SupportWiFiAlpha (Autodesk Fusion 360 design; units mm, degrees)
Autodesk Fusion 360 part; units mm, degrees
note: some values were not read from the file. Chosen so that the rebuilt part matches the saved one: which pieces of a blend or face edit are solid.
sketch "Sketch1" plane through (0, 0, 0) normal (0, 0, 1) x (1, 0, 0)
  line L0 (32.5, -60.9) -> (-32.5, -60.9)
  line L1 (-32.5, -60.9) -> (-32.5, 60.9)
  line L2 (-32.5, 60.9) -> (32.5, 60.9)
  line L3 (32.5, 60.9) -> (32.5, -60.9)
  line L4 (32.5, -60.9) -> (-32.5, 60.9) construction
  line L5 (-32.5, -60.9) -> (32.5, 60.9) construction
  line L6 (0, 0) -> (0, 50.9) construction
  line L7 (-2.1, 52.15) -> (-2.1, 49.65)
  arc A0 (-2.1, 49.65) -> (2.1, 49.65) centre (0, 49.65) ccw
  line L8 (2.1, 49.65) -> (2.1, 52.15)
  arc A1 (2.1, 52.15) -> (-2.1, 52.15) centre (0, 52.15) ccw
  line L9 (0, 52.15) -> (0, 49.65) construction
  line L10 (-32.5, 0) -> (32.5, 0) construction
  arc A2 (-2.1, -52.15) -> (2.1, -52.15) centre (0, -52.15) ccw
  line L11 (-2.1, -52.15) -> (-2.1, -49.65)
  line L12 (2.1, -49.65) -> (2.1, -52.15)
  arc A3 (2.1, -49.65) -> (-2.1, -49.65) centre (0, -49.65) ccw
  line L13 (-31.25, 85) -> (31.25, 85)
  line L14 (31.25, 85) -> (31.25, 0)
  line L15 (31.25, 0) -> (-31.25, 0)
  line L16 (-31.25, 0) -> (-31.25, 85)
  line L17 (-32.5, 60.9) -> (-32.5, 85)
  line L18 (-32.5, 85) -> (-31.25, 85)
  line L19 (32.5, 60.9) -> (32.5, 85)
  line L20 (32.5, 85) -> (31.25, 85)
  line L21 (-32.5, -2) -> (32.5, -2)
  line L22 (-9, 0) -> (9, 0)
  line L23 (9, 0) -> (9, -2)
  line L24 (9, -2) -> (-9, -2)
  line L25 (-9, -2) -> (-9, 0)
  line L26 (0, 85) -> (0, 61) construction
  line L27 (10, 85) -> (-10, 85)
  line L28 (-10, 85) -> (-10, 87)
  line L29 (-10, 87) -> (10, 87)
  line L30 (10, 87) -> (10, 85)
  line L31 (10, 85) -> (-10, 87) construction
  line L32 (-10, 85) -> (10, 87) construction
  line L33 (32.5, 85) -> (-32.5, 85)
  line L34 (-32.5, 85) -> (-32.5, 87)
  line L35 (-32.5, 87) -> (32.5, 87)
  line L36 (32.5, 87) -> (32.5, 85)
  line L37 (32.5, 85) -> (-32.5, 87) construction
  line L38 (-32.5, 85) -> (32.5, 87) construction
  point P0 (0, 50.9)
  point P1 (0, 86)
  point P2 (0, 86)
  dimension "d1" = 121.8
  dimension "d2" = 65
  dimension "d3" = 50.9
  dimension "d4" = 4.2
  dimension "d5" = 2.5
  dimension "d8" = 85
  dimension "d9" = 62.5
  dimension "d10" = 2
  dimension "d13" = 18
  dimension "d14" = 20
  dimension "d15" = 2
  constraint horizontal L0
  constraint perpendicular L0 L1
  constraint parallel L0 L2
  constraint parallel L1 L3
  constraint coincident L4 L6.start
  constraint coincident L5 L6.start
  constraint coincident L6.start origin
  constraint vertical L6
  constraint tangent L7 A0
  constraint tangent A0 L8
  constraint parallel L7 L8
  constraint tangent L8 A1
  constraint tangent L7 A1
  constraint parallel L6 L9
  constraint coincident P0 L6.end
  constraint midpoint L9 P0
  constraint midpoint L1 L10.start
  constraint midpoint L3 L10.end
  constraint symmetric L7.start L10 A2.start
  constraint symmetric L7.end L10 L11.end
  constraint symmetric A0.end L10 L12.start
  constraint symmetric L8.end L10 A2.end
  constraint symmetric A0 L10 A3
  constraint symmetric A1 L10 A2
  constraint horizontal L13
  constraint vertical L14
  constraint horizontal L15
  constraint vertical L16
  constraint midpoint L6.start L15
  constraint perpendicular L2 L17
  constraint perpendicular L16 L18
  constraint perpendicular L2 L19
  constraint perpendicular L14 L20
  constraint coincident L1 L21.start
  constraint coincident L3 L21.end
  constraint perpendicular L3 L21
  constraint horizontal L22
  constraint vertical L23
  constraint horizontal L24
  constraint vertical L25
  constraint midpoint L6.start L22
  constraint coincident L21 L23.end
  constraint midpoint L13 L26.start
  constraint perpendicular L13 L26
  constraint horizontal L27
  constraint perpendicular L27 L28
  constraint parallel L27 L29
  constraint parallel L28 L30
  constraint coincident L31 P2
  constraint coincident L32 P2
  constraint coincident L26 P2
  constraint coincident L13 L27.start
  constraint horizontal L33
  constraint perpendicular L33 L34
  constraint parallel L33 L35
  constraint parallel L34 L36
  constraint coincident L37 P2
  constraint coincident L38 P2
  constraint coincident P2 P1
  measures "d1" distance of L0.end L1.end
  measures "d2" distance of L1.end L2.end
  measures "d3" distance of L6.start P0
  measures "d4" diameter of A0
  measures "d5" distance of A1.centre A0.centre
  measures "d8" distance of L13.start L15.end
  measures "d9" distance of L13.start L13.end
  measures "d10" distance of L10 L21
  measures "d13" distance of L23.end L24.end
  measures "d14" distance of L28.end L29.end
  measures "d15" distance of L27.end L28.end
extrude "Extrude1" add sketch "Sketch1" against normal blind 3
extrude "Extrude2" add sketch "Sketch1" along normal blind 10 contours L2 L3 L14 L15 L21 L23 | L1 L2 L15 L16 L21 L25 | L13 L27 L28 L29 L30 L33 L35
fillet "Fillet4" radius 1.5 1 edges at (-31.25, 0, 5)
fillet "Fillet1" radius 22 2 edges at (32.5, 87, -1.5) (-32.5, 87, -1.5)
fillet "Fillet2" radius 1.5 5 edges at (-31.25, 30.45, 0) (0, 85, 0) (-20.125, 0, 0) (20.125, 0, 0) (31.25, 30.45, 0)
fillet "Fillet3" radius 11 2 edges at (-20.75, -2, 0) (20.75, -2, 0)
named bodies: "Support_WiFi_Alpha"
